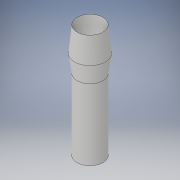
# Autodesk Inventor part: holder thingy
Saved by Autodesk Inventor 2017 (Build 210142000, 142)
## iProperties
Created: 2017-04-26
Part Number: holder thingy
Material: Generic
Document SubType Name: Modeling
Designer: seane
Density: 1 g/cm^3
Appearance: Default
Author: seane
Autodesk Inventor part; units mm, degrees
ref_plane "YZ Plane" through (0, 0, 0) normal (1, 0, 0) x (0, 1, 0)
ref_plane "XZ Plane" through (0, 0, 0) normal (0, 1, 0) x (-1, 0, 0)
ref_plane "XY Plane" through (0, 0, 0) normal (0, 0, 1) x (1, 0, 0)
sketch "Sketch1" plane through (0, 0, 0) normal (1, 0, 0) x (0, 1, 0)
  line L0 (0, 0) -> (0, -12.065)
  line L1 (0, -12.065) -> (91.44, -12.065)
  line L2 (91.44, -12.065) -> (91.44, -13.335)
  line L3 (91.44, -13.335) -> (0, -13.335)
  line L4 (0, -13.335) -> (0, -12.065)
  line L5 (0, 0) -> (110.5631, 0)
  line L6 (91.44, -13.335) -> (116.84, -13.335)
  line L7 (91.44, -13.335) -> (91.44, -15.875)
  line L8 (91.44, -15.875) -> (116.84, -13.335)
  line L9 (91.44, -15.875) -> (73.3806, -13.335)
  dimension "d0" = 12.065
  dimension "d1" = 91.44
  dimension "d2" = 1.27
  dimension "d3" = 25.4
  dimension "d4" = 2.54
  constraints: 20 end point, 4 perpendicular, 2 horizontal, 2 point on line, 2 vertical
  measures "d0" distance of L0.start L0.end
  measures "d1" distance of L0.end L1.end
  measures "d2" distance of L1.end L2.end
  measures "d3" distance of L2.end L6.end
  measures "d4" distance of L2.end L7.end
revolve "Revolution1" add sketch "Sketch1" angle 360 about axis through (0, 0, 0) along (0, 1, 0)
body "Solid1"
